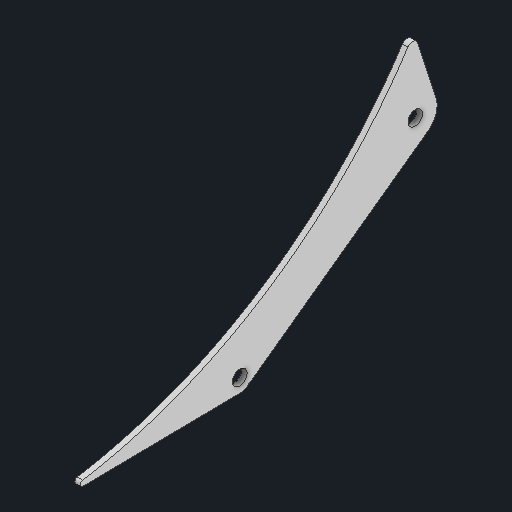
# Autodesk Inventor part: ramp_v3
Saved by Autodesk Inventor 2025 (Build 290162000, 162)
## iProperties
Created: 2024-10-13
Part Number: ramp_v3
Material: Generic
Document SubType Name: Modeling
Designer: Averey Ku
Density: 1 g/cm^3
Appearance: Default
Author: Averey Ku
Autodesk Inventor part; units mm, degrees
ref_plane "YZ Plane" through (0, 0, 0) normal (1, 0, 0) x (0, 1, 0)
ref_plane "XZ Plane" through (0, 0, 0) normal (0, 1, 0) x (-1, 0, 0)
ref_plane "XY Plane" through (0, 0, 0) normal (0, 0, 1) x (1, 0, 0)
sketch "Sketch1" plane through (0, 0, 0) normal (1, 0, 0) x (0, 1, 0)
  circle A0 centre (-23.185, 23.3761) radius 2.1209
  circle A1 centre (16.5025, -27.4239) radius 2.1209 construction
  arc A2 (11.3565, -31.1442) -> (18.4564, -33.4658) centre (16.5025, -27.4239) ccw
  arc A3 (-27.1534, 23.3212) -> (-26.1603, 20.7496) centre (-23.185, 23.3761) ccw
  line L0 (-26.1603, 20.7496) -> (11.3565, -31.1442)
  line L1 (18.4564, -33.4658) -> (34.9319, -28.138)
  arc A4 (34.9319, -28.138) -> (35.3088, -25.2966) centre (34.4434, -26.6275) ccw
  circle A5 centre (16.5025, -27.4239) radius 2.0828
  arc A6 (-26.2045, 68.8566) -> (35.3088, -25.2966) centre (111.6111, 91.725) ccw
  line L2 (-27.7812, 68.7157) -> (-27.1534, 23.3212)
  arc A7 (-26.2045, 68.8566) -> (-27.7812, 68.7157) centre (-26.9875, 68.7267) ccw
  point P0 (0, 0)
  point P1 (-27.9475, 67.8261)
  point P2 (-28.0603, 88.899)
  dimension "d1" = 12.7
  dimension "d5" = 4.1656
  dimension "d6" = 0.7937
  dimension "d7" = 139.7
  constraints: 11 point on circle, 8 centre point, 6 end point, 6 tangent, 3 coincident, 1 point on line, 3 other
  measures "d1" diameter of A2
  measures "d5" diameter of A5
  measures "d6" radius of A7
  measures "d7" radius of A6
extrude "Extrusion1" add sketch "Sketch1" along normal blind 1.5875
body "Solid1"
